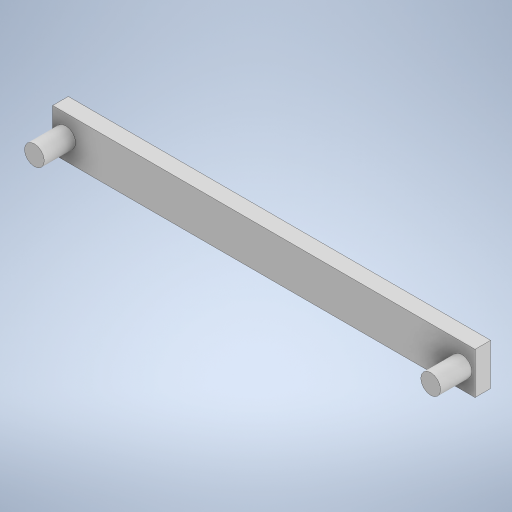
# Autodesk Inventor part: SteeringWheel
Saved by Autodesk Inventor 2024 (Build 280153000, 153)
## iProperties
Created: 2025-12-11
Part Number: SteeringWheel
Material: Generic
Document SubType Name: Modeling
Designer: risda
Density: 1 g/cm^3
Appearance: Default
Author: risda
Autodesk Inventor part; units mm, degrees
ref_plane "YZ Plane" through (0, 0, 0) normal (1, 0, 0) x (0, 1, 0)
ref_plane "XZ Plane" through (0, 0, 0) normal (0, 1, 0) x (-1, 0, 0)
ref_plane "XY Plane" through (0, 0, 0) normal (0, 0, 1) x (1, 0, 0)
sketch "Sketch1" plane through (0, 0, 0) normal (0, 0, 1) x (1, 0, 0)
  line L0 (0, 0) -> (76, 0)
  line L1 (76, 0) -> (76, -8)
  line L2 (76, -8) -> (0, -8)
  line L3 (0, -8) -> (0, 0)
  dimension "d0" = 76
  dimension "d1" = 8
  constraints: 8 end point, 2 perpendicular, 1 horizontal, 1 vertical
  measures "d0" distance of L0.start L0.end
  measures "d1" distance of L0.end L1.end
extrude "Extrusion1" add sketch "Sketch1" along normal blind 3
sketch "Sketch2" plane through (0, 0, 3) normal (0, 0, 1) x (1, 0, 0)
  line L0 (0, 0) -> (0, -8) projected
  circle A0 centre (0, -4) radius 1.9
  line L1 (76, -8) -> (76, 0) projected
  circle A1 centre (76, -4) radius 1.9
  dimension "d4" = 3.8
  dimension "d5" = 3.8
  constraints: 2 centre point, 2 midpoint
  measures "d4" diameter of A0
  measures "d5" diameter of A1
extrude "Extrusion2" add sketch "Sketch2" along normal blind 6
sketch "Sketch3" plane through (0, 0, 0) normal (0, 0, -1) x (-1, 0, 0)
  line L0 (0, -8) -> (-76, -8) projected
  line L1 (0, -8) -> (2.5, -8)
  line L2 (2.5, -8) -> (2.5, 0)
  line L3 (2.5, 0) -> (0, 0)
  line L4 (0, 0) -> (0, -8)
  line L5 (-76, -8) -> (-78.5, -8)
  line L6 (-78.5, -8) -> (-78.5, 0)
  line L7 (-78.5, 0) -> (-76, 0)
  line L8 (-76, 0) -> (-76, -8)
  dimension "d8" = 2.5
  dimension "d9" = 2.5
  constraints: 16 end point, 4 parallel, 2 horizontal, 2 perpendicular
  measures "d8" distance of L3.end L2.end
  measures "d9" distance of L6.end L7.end
extrude "Extrusion3" add sketch "Sketch3" against normal blind 3
body "Solid1"
